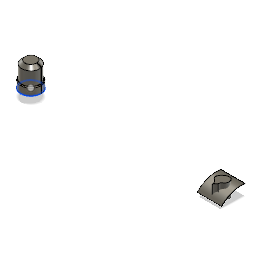
6.1 boolean (Autodesk Fusion 360 design; units mm, degrees)
Autodesk Fusion 360 part; units mm, degrees
sketch "Sketch1" plane through (0, 0, 0) normal (0, 1, 0) x (1, 0, 0)
  spline S0 degree 5 poles (0, 0) (0.0619, 1.1722) (0.0831, 3.4699) (-0.1929, 6.7763) (-1.1772, 10.9043) (-3.4126, 15.6061) (-6.576, 19.8821) (-10.5098, 23.799) (-14.9381, 27.4739) (-19.4646, 31.0742) (-23.6399, 34.7853) (-27.0158, 38.784) (-29.2005, 43.2113) (-29.924, 48.1422) (-29.0612, 53.5689) (-26.6045, 59.4018) (-22.6508, 65.4644) (-17.3842, 71.4924) (-11.0602, 77.1242) (-3.9899, 81.916) (3.4782, 85.4117) (10.9753, 87.2028) (18.13, 86.9915) (24.5856, 84.6553) (30.0175, 80.3073) (34.1503, 74.3713) (36.7795, 67.4723) (37.7922, 60.3152) (37.19, 53.565) (35.109, 47.7341) (31.85, 43.0476) (27.8797, 39.3735) (23.7418, 36.367) (19.9788, 33.5816) (17.0583, 30.5831) (15.2775, 27.0863) (14.8757, 23.7837) (15.1697, 21.0022) (15.6298, 19.0128) (15.926, 17.9844) knots 0 0 0 0 0 0 0.028571 0.057143 0.085714 0.114286 0.142857 0.171429 0.2 0.228571 0.257143 0.285714 0.314286 0.342857 0.371429 0.4 0.428571 0.457143 0.485714 0.514286 0.542857 0.571429 0.6 0.628571 0.657143 0.685714 0.714286 0.742857 0.771429 0.8 0.828571 0.857143 0.885714 0.914286 0.942857 0.971429 1 1 1 1 1 1
  arc A0 (15.926, 17.9844) -> (0, 0) centre (37.8656, -17.4879) ccw
  point P0 (-9.2465, 22.4266)
  point P1 (-28.0025, 41.1826)
  point P2 (-18.8713, 69.5633)
  point P3 (24.8104, 83.8771)
  point P4 (35.4223, 49.3266)
  point P5 (19.1342, 32.545)
  constraint coincident S0.start A0.end
sketch "Sketch2" plane through (0, 0, 0) normal (1, 0, 0) x (0, 0, -1)
  line L0 (0, 0) -> (86.853, 0)
  arc A0 (121.9894, 21.3126) -> (-17.4465, -25.0838) centre (93.7289, -126.4784) ccw
  arc A1 (121.5535, 19.0328) -> (-15.7315, -26.6478) centre (93.7289, -126.4784) ccw
  line L1 (-17.4465, -25.0838) -> (-15.7315, -26.6478)
  line L2 (121.5535, 19.0328) -> (121.9894, 21.3126)
  dimension "d1" = -2.3211
extrude "Extrude1" add sketch "Sketch1" along normal mid plane 86.62 makes body 1
extrude "Extrude2" add sketch "Sketch2" along normal mid plane 142.432 separate body makes body 2
sketch "Sketch3" plane through (0, 0, 0) normal (0, 1, 0) x (1, 0, 0)
  circle A0 centre (-1055.8026, 0.0288) radius 52.5067
  circle A1 centre (-1055.8026, 0.0288) radius 59.1357
  constraint concentric A0 A1
extrude "Extrude3" add sketch "Sketch3" along normal blind 141.726 separate body contours A0 makes body 3
extrude "Extrude4" add sketch "Sketch3" along normal blind 44.464 bodies 3
fillet "Fillet1" radius 3.809 1 edges at (-1110.9365, 44.464, 21.3556) on bodies 3
chamfer "Chamfer1" distance 18.82 angle 45 1 edges at (-1104.7561, 141.726, 18.9585) on bodies 3
sketch "Sketch4" plane through (0, 141.726, 0) normal (0, 1, 0) x (-1, 0, 0)
  circle A0 centre (1055.8026, -0.0288) radius 33.6867
  line L0 (1024.6879, 0.8425) -> (993.8479, 0.8425)
  line L1 (993.8479, 0.8425) -> (993.8479, -0.7775)
  line L2 (993.8479, -0.7775) -> (1024.6879, -0.7775)
  line L3 (1024.6879, -0.7775) -> (1024.6879, 0.8425)
  circle A1 centre (1055.8026, -0.0288) radius 52.5067
  constraint horizontal L0
  constraint horizontal L2
  constraint vertical L3
  constraint coincident L1.end L2.start
extrude "Extrude5" add sketch "Sketch4" against normal up to surface (141.726 mm away) separate body contours A0 L0 L2 A1 | L0 L1 L2 A1 picked at (1015.8474, -0.5975) makes body 4
fillet "Fillet2" radius 18.579 1 edges at (-993.8479, 141.726, 0.0325) on bodies 4
named bodies: "Blade flat", "Blade arc", "Knob body", "Knob fin"
